spiceholder (Autodesk Fusion 360 design; units mm, degrees)
Autodesk Fusion 360 part; units mm, degrees
sketch "Sketch1" plane through (0, 0, 0) normal (0, 1, 0) x (1, 0, 0)
  circle A0 centre (0, 0) radius 1
  dimension "d1" = 2
  constraint coincident A0.centre origin
  measures "d1" diameter of A0
extrude "Extrude1" add sketch "Sketch1" along normal blind 240 and the other way blind 10 makes body 1
pattern_linear "R-Pattern1" count 13 spacing 27.0833 along (1, 0, 0) of bodies 1 makes body 2 at (26.718, 160, 0.9309) makes body 3 at (54.8997, 160, -0.6802) makes body 4 at (81.1753, 160, -0.9972) makes body 5 at (108.2586, 160, -0.9972) makes body 6 at (135.0513, 160, 0.9309) makes body 7 at (162.1347, 160, 0.9309) makes body 8 at (189.218, 160, 0.9309) makes body 9 at (216.3013, 160, 0.9309) makes body 10 at (243.3847, 160, 0.9309) makes body 11 at (270.7586, 160, -0.9972) makes body 12 at (297.8419, 160, -0.9972) makes body 13 at (324.9253, 160, -0.9972)
sketch "Sketch2" plane through (0, 0, 0) normal (1, 0, 0) x (0, 1, 0)
  circle A0 centre (0, -2) radius 1
  line L0 (0, 0) -> (0, -2)
  dimension "d8" = 2
  dimension "d9" = 2
  constraint coincident L0.start origin
  constraint vertical L0
  constraint coincident A0.centre L0.end
  measures "d8" diameter of A0
  measures "d9" distance of L0.start A0.centre
extrude "Extrude2" add sketch "Sketch2" along normal blind 340 and the other way blind 10 separate body makes body 14
pattern_linear "R-Pattern2" count 10 spacing 27.0556 along (0, 1, 0) of bodies 14 makes body 15 at (226.6667, 26.1546, -1.5661) makes body 16 at (226.6667, 53.2101, -1.5661) makes body 17 at (226.6667, 80.5432, -2.7818) makes body 18 at (226.6667, 107.5987, -2.7818) makes body 19 at (113.3333, 135.0553, -1.0251) makes body 20 at (113.3333, 162.1108, -1.0251) makes body 21 at (113.3333, 189.1664, -1.0251) makes body 22 at (113.3333, 216.2219, -1.0251) makes body 23 at (113.3333, 243.2775, -1.0251)
sketch "Sketch3" plane through (0, 0, 0) normal (0, 0, 1) x (1, 0, 0)
  circle A0 centre (15, 15) radius 24
  circle A1 centre (15, 15) radius 22.5
  line L0 (15, 15) -> (-9, 15) construction
  line L1 (15, 15) -> (15, -9) construction
  circle A2 centre (15, 62.5) radius 22.5
  circle A3 centre (15, 62.5) radius 24
  circle A4 centre (15, 110) radius 22.5
  circle A5 centre (15, 110) radius 24
  circle A6 centre (15, 157.5) radius 22.5
  circle A7 centre (15, 157.5) radius 24
  circle A8 centre (15, 205) radius 22.5
  circle A9 centre (15, 205) radius 24
  line L2 (15, 205) -> (-9, 205)
  line L3 (15, 205) -> (15, 229)
  line L4 (-9, 205) -> (-9, 15)
  line L5 (15, 205) -> (-1.9706, 188.0294)
  line L6 (15, 15) -> (-1.9706, 31.9706) construction
  line L7 (-1.9706, 188.0294) -> (-1.9706, 31.9706)
  circle A10 centre (64.1667, 205) radius 24
  circle A11 centre (64.1667, 205) radius 22.5
  circle A12 centre (64.1667, 157.5) radius 24
  circle A13 centre (64.1667, 157.5) radius 22.5
  circle A14 centre (64.1667, 110) radius 24
  circle A15 centre (64.1667, 110) radius 22.5
  circle A16 centre (64.1667, 62.5) radius 24
  circle A17 centre (64.1667, 62.5) radius 22.5
  circle A18 centre (64.1667, 15) radius 24
  circle A19 centre (64.1667, 15) radius 22.5
  circle A20 centre (113.3333, 205) radius 24
  circle A21 centre (113.3333, 205) radius 22.5
  circle A22 centre (113.3333, 157.5) radius 24
  circle A23 centre (113.3333, 157.5) radius 22.5
  circle A24 centre (113.3333, 110) radius 24
  circle A25 centre (113.3333, 110) radius 22.5
  circle A26 centre (113.3333, 62.5) radius 24
  circle A27 centre (113.3333, 62.5) radius 22.5
  circle A28 centre (113.3333, 15) radius 24
  circle A29 centre (113.3333, 15) radius 22.5
  circle A30 centre (162.5, 205) radius 24
  circle A31 centre (162.5, 205) radius 22.5
  circle A32 centre (162.5, 157.5) radius 24
  circle A33 centre (162.5, 157.5) radius 22.5
  circle A34 centre (162.5, 110) radius 24
  circle A35 centre (162.5, 110) radius 22.5
  circle A36 centre (162.5, 62.5) radius 24
  circle A37 centre (162.5, 62.5) radius 22.5
  circle A38 centre (162.5, 15) radius 24
  circle A39 centre (162.5, 15) radius 22.5
  circle A40 centre (211.6667, 205) radius 24
  circle A41 centre (211.6667, 205) radius 22.5
  circle A42 centre (211.6667, 157.5) radius 24
  circle A43 centre (211.6667, 157.5) radius 22.5
  circle A44 centre (211.6667, 110) radius 24
  circle A45 centre (211.6667, 110) radius 22.5
  circle A46 centre (211.6667, 62.5) radius 24
  circle A47 centre (211.6667, 62.5) radius 22.5
  circle A48 centre (211.6667, 15) radius 24
  circle A49 centre (211.6667, 15) radius 22.5
  circle A50 centre (260.8333, 205) radius 24
  circle A51 centre (260.8333, 205) radius 22.5
  circle A52 centre (260.8333, 157.5) radius 24
  circle A53 centre (260.8333, 157.5) radius 22.5
  circle A54 centre (260.8333, 110) radius 24
  circle A55 centre (260.8333, 110) radius 22.5
  circle A56 centre (260.8333, 62.5) radius 24
  circle A57 centre (260.8333, 62.5) radius 22.5
  circle A58 centre (260.8333, 15) radius 24
  circle A59 centre (260.8333, 15) radius 22.5
  circle A60 centre (310, 205) radius 24
  circle A61 centre (310, 205) radius 22.5
  circle A62 centre (310, 157.5) radius 24
  circle A63 centre (310, 157.5) radius 22.5
  circle A64 centre (310, 110) radius 24
  circle A65 centre (310, 110) radius 22.5
  circle A66 centre (310, 62.5) radius 24
  circle A67 centre (310, 62.5) radius 22.5
  circle A68 centre (310, 15) radius 24
  circle A69 centre (310, 15) radius 22.5
  line L8 (15, 15) -> (30.9099, -0.9099) construction
  line L9 (310, 15) -> (294.0901, -0.9099)
  line L10 (310, 15) -> (325.9099, 30.9099)
  line L11 (310, 205) -> (325.9099, 189.0901)
  line L12 (310, 205) -> (294.0901, 220.9099)
  line L13 (15, 205) -> (30.9099, 220.9099)
  line L14 (310, 15) -> (310, -9)
  line L15 (310, 15) -> (334, 15)
  line L16 (310, 205) -> (310, 229)
  line L17 (310, 205) -> (286, 205)
  line L18 (310, 205) -> (310, 181)
  line L19 (30.9099, 220.9099) -> (31.9706, 221.9706)
  line L20 (31.9706, 221.9706) -> (293.0294, 221.9706)
  line L21 (294.0901, 220.9099) -> (293.0294, 221.9706)
  line L22 (325.9099, 189.0901) -> (326.9706, 188.0294)
  line L23 (326.9706, 188.0294) -> (326.9706, 31.9706)
  line L24 (325.9099, 30.9099) -> (326.9706, 31.9706)
  line L25 (294.0901, -0.9099) -> (293.0294, -1.9706)
  line L26 (293.0294, -1.9706) -> (31.9706, -1.9706)
  line L27 (31.9706, -1.9706) -> (30.9099, -0.9099) construction
  dimension "d20" = 48
  dimension "d21" = 15
  dimension "d22" = 15
  dimension "d23" = 45
  dimension "d29" = 0
  dimension "d30" = 190
  dimension "d31" = 45
  dimension "d32" = 45
  dimension "d35" = 295
  dimension "d36" = 0
  dimension "d37" = 45
  dimension "d38" = 45
  dimension "d39" = 45
  dimension "d40" = 45
  dimension "d41" = 45
  constraint concentric A0 A1
  constraint coincident A0.centre A1.centre
  constraint coincident A0 L0.end
  constraint horizontal L0
  constraint coincident A0 L1.end
  constraint perpendicular L0 L1
  constraint coincident A8.centre A9.centre
  constraint coincident A9 L2.end
  constraint horizontal L2
  constraint coincident A9 L3.end
  constraint perpendicular L2 L3
  constraint coincident A9 L5.end
  constraint coincident A0 L6.end
  constraint coincident A1 L8.end
  constraint coincident A68.centre A69.centre
  constraint coincident A69 L9.end
  constraint coincident A69 L10.end
  constraint parallel L9 L10
  constraint coincident A60.centre A61.centre
  constraint coincident A61 L11.end
  constraint coincident A61 L12.end
  constraint coincident A8 L13.end
  constraint coincident A68 L14.end
  constraint vertical L14
  constraint coincident A68 L15.end
  constraint horizontal L15
  constraint coincident A60 L16.end
  constraint perpendicular L15 L16
  constraint coincident A60 L17.end
  constraint perpendicular L16 L17
  constraint coincident A60 L18.end
  constraint vertical L18
  constraint coincident A9 L19.end
  constraint parallel L13 L19
  constraint coincident A60 L20.end
  constraint horizontal L20
  constraint coincident A60 L22.end
  constraint parallel L11 L22
  constraint coincident A68 L23.end
  constraint vertical L23
  constraint coincident L10 L24.start
  constraint coincident L10.end L24.start
  constraint coincident A68 L25.end
  constraint parallel L9 L25
  constraint coincident A0 L26.end
  constraint horizontal L26
  measures "d20" diameter of A0
  measures "d21" horizontal distance of origin A0.centre
  measures "d22" vertical distance of origin A0.centre
  measures "d23" diameter of A1
  measures "d31" angle of L0 L6
  measures "d32" angle of L2 L5
  measures "d37" angle of L3 L13
  measures "d38" angle of L1 L8
  measures "d39" angle of L12 L17
  measures "d40" angle of L11 L18
  measures "d41" angle of L10 L15
extrude "Extrude1'" add sketch "Sketch3" along normal blind 45 from surface at 1 separate body contours A0 A3 | A0 A3 L7 | A0 A2 A3 A5 L7 | A0 A3 | A2 A3 L7 | A0 A3 A5 A7 A9 A10 A12 A14 A16 A18 L20 L26 | A18 A19 L26 | A16 A18 A19 L26 | A3 A5 L7 | A4 A5 L7 | A16 A18 | A14 A16 A18 | A10 A12 A14 A16 A18 A20 A22 A24 A26 A28 L20 L26 | A3 A4 A5 A7 L7 | A3 A5 | A5 A7 L7 | A6 A7 L7 | A14 A16 | A12 A14 A16 | A28 A29 L26 | A26 A28 A29 L26 | A5 A6 A7 A9 L7 | A5 A7 | A7 A9 L7 | A8 A9 L2 L5 | A8 A9 L2 L3 | A12 A14 | A10 A12 A14 | A26 A28 | A24 A26 A28 | A20 A22 A24 A26 A28 A30 A32 A34 A36 A38 L20 L26 | A7 A8 A9 L5 L19 | A7 A9 | A8 A9 L3 L19 | A10 A12 | A10 A11 A12 L20 | A24 A26 | A22 A24 A26 | A38 A39 L26 | A36 A38 A39 L26 | A10 A11 L20 | A22 A24 | A20 A22 A24 | A36 A38 | A34 A36 A38 | A30 A32 A34 A36 A38 A40 A42 A44 A46 A48 L20 L26 | A20 A22 | A20 A21 A22 L20 | A34 A36 | A32 A34 A36 | A48 A49 L26 | A46 A48 A49 L26 | A20 A21 L20 | A32 A34 | A30 A32 A34 | A46 A48 | A44 A46 A48 | A40 A42 A44 A46 A48 A50 A52 A54 A56 A58 L20 L26 | A30 A32 | A30 A31 A32 L20 | A44 A46 | A42 A44 A46 | A58 A59 L26 | A56 A58 A59 L26 | A30 A31 L20 | A42 A44 | A40 A42 A44 | A56 A58 | A54 A56 A58 | A50 A52 A54 A56 A58 A60 A62 A64 A66 A68 L20 L26 | A40 A42 | A40 A41 A42 L20 | A54 A56 | A52 A54 A56 | A68 A69 L14 L25 | A66 A68 A69 L24 L25 | A40 A41 L20 | A52 A54 | A50 A52 A54 | A68 A69 L14 L15 | A66 A68 | A64 A66 A67 A68 L23 | A50 A52 | A50 A51 A52 L20 | A68 A69 L15 L24 | A64 A66 | A62 A64 A65 A66 L23 | A66 A68 L23 | A50 A51 L20 | A62 A64 | A60 A62 A63 A64 L23 | A64 A66 L23 | A66 A67 L23 | A60 A62 L18 | A60 A61 A62 L17 L18 | A64 A65 L23 | A60 A61 L17 L21 | A60 A61 L16 L21 | A60 A62 L18 | A60 A61 A62 L18 L22 | A62 A63 L23 | A60 A61 L16 L22 | A60 A62 L23 makes body 24 in component "Component"
extrude "Extrude2'" add 1 faces at (283.0788, 41.1986, 1) along direction (0, 0, -1) blind 4 on bodies 24 bodies 24 in component "Component"
combine "Combine1" operation cut target body 24 tool bodies 16 13 15 17 18 19 20 21 22 14 1 2 3 4 5 6 7 8 9 10 12 11 keep tools in component "Component"
sketch "Sketch4" plane through (0, -1.9706, 0) normal (0, -1, 0) x (1, 0, 0)
  line L0 (47.1961, -3) -> (47.1961, 46)
  line L1 (47.1961, 46) -> (31.9706, 46)
  line L2 (31.9706, 46) -> (31.9706, -3)
  line L3 (31.9706, -3) -> (47.1961, -3)
  line L4 (-1, 0) -> (1, 0)
  line L5 (1, 0) -> (1, -5)
  line L6 (1, -5) -> (-1, -5)
  line L7 (-1, -5) -> (-1, 0)
  circle A0 centre (0, 0) radius 1
  line L8 (-1, 0) -> (1, 0)
  circle A1 centre (0, 0) radius 1.1
  line L9 (1.1, 0) -> (-1.1, 0)
  line L10 (1.1, 0) -> (-1.1, 0)
  line L11 (-1.1, 0) -> (-1.1, -5)
  line L12 (-1.1, -5) -> (1.1, -5)
  line L13 (1.1, -5) -> (1.1, 0)
  point P0 (-1, 0)
  dimension "d44" = 2
  dimension "d45" = 5
  dimension "d67" = 0.1
  constraint horizontal L4
  constraint vertical L5
  constraint horizontal L6
  constraint vertical L7
  constraint coincident A0.centre A1.centre
  constraint coincident L4.end A0
  constraint coincident L7 P0
  constraint coincident P0 L4.start
  constraint coincident A1 L9.start
  constraint coincident A1 L9.end
  constraint perpendicular L7 L9
  constraint horizontal L10
  constraint vertical L11
  constraint horizontal L12
  constraint vertical L13
  constraint tangent A1 L11
  constraint tangent A1 L13
  measures "d44" diameter of A0
  measures "d45" distance of L4.end L5.end
  measures "d67" distance of A0 A1
extrude "Extrude3" [suppressed]
extrude "Extrude3'" cut sketch "Sketch4" along normal mid plane 483.9411 contours L4 A0 L8 L9 L10 | L5 L7 A0 A1 | A0 A1 L9 L10 | L4 A0 L8 L9 L10 | L7 A1 L9 L10 | L5 A1 L9 L10 | L5 L6 L7 A1 L12 | L7 A1 L11 L12 | L5 A1 L12 L13 bodies 24 in component "Component"
pattern_linear "R-Pattern3" [no effect]
pattern_linear "R-Pattern1'" count 13 spacing 27.0833 along (1, 0, 0) of "Extrude3'" in component "Component"
sketch "Sketch5" plane through (340, 0, 0) normal (1, 0, 0) x (0, 1, 0)
  circle A0 centre (0, -2) radius 1
  line L0 (-1, -2) -> (1, -2)
  line L1 (1, -2) -> (1, -7)
  line L2 (1, -7) -> (-1, -7)
  line L3 (-1, -7) -> (-1, -2)
  circle A1 centre (0, -2) radius 1
  circle A2 centre (0, -2) radius 1.15
  line L4 (1.15, -2) -> (-1.15, -2)
  line L5 (-1.15, -2) -> (-1.15, -7.5)
  line L6 (-1.15, -7.5) -> (1.15, -7.5)
  line L7 (1.15, -7.5) -> (1.15, -2)
  dimension "d58" = 5
  dimension "d68" = 0.15
  constraint horizontal L0
  constraint vertical L1
  constraint horizontal L2
  constraint vertical L3
  constraint coincident A0 L0.start
  constraint concentric A0 A1
  constraint equal A0 A1
  constraint coincident L0.end A1
  constraint coincident L0 A0.centre
  constraint concentric A1 A2
  constraint horizontal L4
  constraint vertical L5
  constraint horizontal L6
  constraint vertical L7
  constraint coincident A0.centre L4
  constraint tangent A2 L5
  constraint tangent A2 L7
  measures "d58" distance of L0.end L1.end
  measures "d68" distance of A1 A2
extrude "Extrude4" cut sketch "Sketch5" against normal blind 400 bodies 24 in component "Component"
pattern_linear "R-Pattern2'" count 10 spacing 27.0556 along (0, 1, 0) of "Extrude4" in component "Component"
chamfer "Chamfer1" distance 1.5 distance2 10 35 edges at (289.0226, 23.1363, 46) (289.0226, 70.6363, 46) (289.0226, 118.1363, 46) (289.0226, 165.6363, 46) (239.856, 118.1363, 46) (239.856, 70.6363, 46) (239.856, 23.1363, 46) (239.856, 165.6363, 46) (239.856, 213.1363, 46) (289.0226, 213.1363, 46) (190.6893, 23.1363, 46) (141.5226, 23.1363, 46) (141.5226, 70.6363, 46) (190.6893, 70.6363, 46) (190.6893, 118.1363, 46) (141.5226, 118.1363, 46) (190.6893, 165.6363, 46) (141.5226, 165.6363, 46) (141.5226, 213.1363, 46) (190.6893, 213.1363, 46) (92.356, 213.1363, 46) (92.356, 165.6363, 46) (92.356, 118.1363, 46) (92.356, 70.6363, 46) (92.356, 23.1363, 46) (43.1893, 23.1363, 46) (-5.9774, 23.1363, 46) (-5.9774, 70.6363, 46) (43.1893, 70.6363, 46) (-5.9774, 118.1363, 46) (43.1893, 118.1363, 46) (43.1893, 165.6363, 46) (-5.9774, 165.6363, 46) (-5.9774, 213.1363, 46) (43.1893, 213.1363, 46) measured on face at (283.0383, 178.7574, 46) measured on face at (283.0383, 178.7574, 46) measured on face at (283.0383, 178.7574, 46) measured on face at (283.0383, 178.7574, 46) measured on face at (283.0383, 178.7574, 46) measured on face at (283.0383, 178.7574, 46) measured on face at (283.0383, 178.7574, 46) measured on face at (283.0383, 178.7574, 46) measured on face at (283.0383, 178.7574, 46) measured on face at (283.0383, 178.7574, 46) measured on face at (283.0383, 178.7574, 46) measured on face at (283.0383, 178.7574, 46) measured on face at (283.0383, 178.7574, 46) measured on face at (283.0383, 178.7574, 46) measured on face at (283.0383, 178.7574, 46) measured on face at (283.0383, 178.7574, 46) measured on face at (283.0383, 178.7574, 46) measured on face at (283.0383, 178.7574, 46) measured on face at (283.0383, 178.7574, 46) measured on face at (283.0383, 178.7574, 46) measured on face at (283.0383, 178.7574, 46) measured on face at (283.0383, 178.7574, 46) measured on face at (283.0383, 178.7574, 46) measured on face at (283.0383, 178.7574, 46) measured on face at (283.0383, 178.7574, 46) measured on face at (283.0383, 178.7574, 46) measured on face at (283.0383, 178.7574, 46) measured on face at (283.0383, 178.7574, 46) measured on face at (283.0383, 178.7574, 46) measured on face at (283.0383, 178.7574, 46) measured on face at (283.0383, 178.7574, 46) measured on face at (283.0383, 178.7574, 46) measured on face at (283.0383, 178.7574, 46) measured on face at (283.0383, 178.7574, 46) measured on face at (283.0383, 178.7574, 46) on bodies 24 in component "Component"
component "Component" placed x (1, 0, 0) y (0, 1, 0) z (0, 0, 1) at (0, 0, 0)
equation "d6 = ( 13 * 25 ) * 1 mm"
